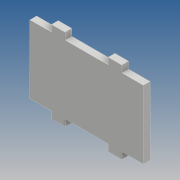
# Autodesk Inventor part: Ball Capture Zone Cover plate
Saved by Autodesk Inventor 2017 (Build 210142000, 142)
## iProperties
Created: 2017-06-26
Part Number: Ball Capture Zone Cover plate
Material: Generic
Document SubType Name: Modeling
Designer: yella
Density: 1 g/cm^3
Appearance: Default
Author: yella
Autodesk Inventor part; units mm, degrees
ref_plane "YZ Plane" through (0, 0, 0) normal (1, 0, 0) x (0, 1, 0)
ref_plane "XZ Plane" through (0, 0, 0) normal (0, 1, 0) x (-1, 0, 0)
ref_plane "XY Plane" through (0, 0, 0) normal (0, 0, 1) x (1, 0, 0)
sketch "Sketch1" plane through (0, 0, 0) normal (0, 1, 0) x (-1, 0, 0)
  line L0 (-15.5, 0) -> (-15.5, 3)
  line L1 (-15.5, 3) -> (-9.5, 3)
  line L2 (-9.5, 3) -> (-9.5, 0)
  line L3 (15.5, 0) -> (15.5, 3)
  line L4 (15.5, 3) -> (9.5, 3)
  line L5 (9.5, 3) -> (9.5, 0)
  line L6 (-15.5, 0) -> (-15.5, 3)
  line L7 (-15.5, 3) -> (-9.5, 3)
  line L8 (-9.5, 3) -> (-9.5, 0)
  line L9 (15.5, 0) -> (15.5, 3)
  line L10 (15.5, 3) -> (9.5, 3)
  line L11 (9.5, 3) -> (9.5, 0)
  line L12 (-25, 0) -> (-15.5, 0)
  line L13 (-9.5, 0) -> (9.5, 0)
  line L14 (15.5, 0) -> (25, 0)
  line L15 (25, 0) -> (25, -30)
  line L16 (-25, 0) -> (-25, -30)
  line L17 (25, -30) -> (15.5, -30)
  line L18 (15.5, -30) -> (15.5, -33)
  line L19 (15.5, -33) -> (9.5, -33)
  line L20 (9.5, -33) -> (9.5, -30)
  line L21 (9.5, -30) -> (-9.5, -30)
  line L22 (-9.5, -30) -> (-9.5, -33)
  line L23 (-9.5, -33) -> (-15.5, -33)
  line L24 (-15.5, -33) -> (-15.5, -30)
  line L25 (-15.5, -30) -> (-25, -30)
  point P0 (0, 0)
  dimension "d3" = 3
  dimension "d4" = 6
  dimension "d7" = 3
  dimension "d8" = 6
  dimension "d12" = 3
  dimension "d13" = 6
  dimension "d16" = 3
  dimension "d17" = 6
  dimension "d19" = 30
  dimension "d20" = 30
  dimension "d21" = 3
  constraints: 52 end point, 11 perpendicular, 5 point on line, 1 horizontal, 1 vertical
  measures "d3" distance of L0.start L0.end
  measures "d4" distance of L0.end L1.end
  measures "d7" distance of L3.start L3.end
  measures "d8" distance of L3.end L4.end
  measures "d12" distance of L6.start L6.end
  measures "d13" distance of L6.end L8.start
  measures "d16" distance of L9.start L9.end
  measures "d17" distance of L9.end L10.end
  measures "d19" distance of L12.start L16.end
  measures "d20" distance of L14.end L15.end
  measures "d21" distance of L17.end L18.end
extrude "Extrusion1" add sketch "Sketch1" along normal blind 3
body "Solid1"
